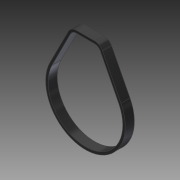
# Autodesk Inventor part: Weight Shifter Tension Strap
Saved by Autodesk Inventor 2014 SP1 (Build 180222100, 222)
## iProperties
Created: 2013-12-18
Part Number: Weight Shifter Tension Strap
Material: Rubber
Document SubType Name: Modeling
Designer: Moses
Density: 0.93 g/cm^3
Appearance: Rubber - Black - Version 1.1
Mass: 6.13624 g
Surface Area: 66.1476 cm^2
Volume: 6.59811 cm^3
Author: Moses
Autodesk Inventor part; units mm, degrees
ref_plane "YZ Plane" through (0, 0, 0) normal (1, 0, 0) x (0, 1, 0)
ref_plane "XZ Plane" through (0, 0, 0) normal (0, 1, 0) x (-1, 0, 0)
ref_plane "XY Plane" through (0, 0, 0) normal (0, 0, 1) x (1, 0, 0)
sketch "Sketch1" plane through (0, 0, 0) normal (0, 0, 1) x (1, 0, 0)
  arc A0 (-26.9408, 26.9408) -> (26.9408, 26.9408) centre (0, 0) ccw construction
  line L0 (-15.875, 29.0994) -> (-12.7, 29.0994) construction
  line L1 (-15.875, 51.3244) -> (-15.875, 29.0994) construction
  arc A1 (-9.525, 57.6744) -> (-15.875, 51.3244) centre (-9.525, 51.3244) ccw construction
  line L2 (9.525, 57.6744) -> (-9.525, 57.6744) construction
  arc A2 (15.875, 51.3244) -> (9.525, 57.6744) centre (9.525, 51.3244) ccw construction
  line L3 (15.875, 29.0994) -> (15.875, 51.3244) construction
  line L4 (12.7, 29.0994) -> (15.875, 29.0994) construction
  line L5 (12.7, 51.3244) -> (12.7, 29.0994) construction
  arc A3 (12.7, 51.3244) -> (9.525, 54.4994) centre (9.525, 51.3244) ccw construction
  line L6 (-9.525, 54.4994) -> (9.525, 54.4994) construction
  arc A4 (-9.525, 54.4994) -> (-12.7, 51.3244) centre (-9.525, 51.3244) ccw construction
  line L7 (-12.7, 29.0994) -> (-12.7, 51.3244) construction
  line L8 (-33.963, 17.2662) -> (-15.1855, 54.2021)
  line L9 (33.963, 17.2662) -> (15.1855, 54.2021)
  arc A5 (-9.525, 57.6744) -> (-15.1855, 54.2021) centre (-9.525, 51.3244) ccw
  arc A6 (15.1855, 54.2021) -> (9.525, 57.6744) centre (9.525, 51.3244) ccw
  line L10 (-9.525, 57.6744) -> (9.525, 57.6744)
  arc A7 (-33.963, 17.2662) -> (33.963, 17.2662) centre (0, 0) ccw
  line L11 (-17.4497, 55.3531) -> (-36.2272, 18.4173)
  arc A8 (-36.2272, 18.4173) -> (36.2272, 18.4173) centre (0, 0) ccw
  line L12 (36.2272, 18.4173) -> (17.4497, 55.3531)
  arc A9 (17.4497, 55.3531) -> (9.525, 60.2144) centre (9.525, 51.3244) ccw
  line L13 (9.525, 60.2144) -> (-9.525, 60.2144)
  arc A10 (-9.525, 60.2144) -> (-17.4497, 55.3531) centre (-9.525, 51.3244) ccw
  point P0 (0, 0)
  dimension "d0" = 2.54
  constraints: 16 point on circle, 12 end point, 12 tangent, 6 centre point, 2 concentric, 1 horizontal, 5 other
  measures "d0" distance between parallel lines of L13 L10
extrude "Extrusion1" add sketch "Sketch1" along normal blind 9.297
body "Solid1"
